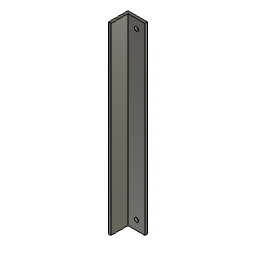
angle iron 1 inch 240 mm v12 (Autodesk Fusion 360 design; units mm, degrees)
Autodesk Fusion 360 part; units mm, degrees
sketch "Sketch1" plane through (0, 0, 0) normal (0, 0, 1) x (1, 0, 0)
  line L0 (0, 0) -> (25.4, 0)
  line L1 (0, 0) -> (0, -25.4)
  line L2 (3.175, -3.175) -> (25.4, -3.175)
  line L3 (3.175, -3.175) -> (3.175, -25.4)
  line L4 (25.4, 0) -> (25.4, -3.175)
  line L5 (0, -25.4) -> (3.175, -25.4)
  dimension "d1" = 25.4
  dimension "d2" = -3.175
  constraint coincident L0.start L1.start
  constraint horizontal L0
  constraint perpendicular L0 L1
  constraint equal L0 L1
  measures "d1" distance of L0.start L0.end
extrude "Extrude1" add sketch "Sketch1" along normal blind 240
sketch "Sketch2" plane through (0, -3.175, 0) normal (0, -1, 0) x (1, 0, 0)
  line L0 (3.175, 0) -> (25.4, 0)
  line L1 (25.4, 0) -> (25.4, 240)
  line L2 (25.4, 240) -> (3.175, 240)
  line L3 (3.175, 240) -> (3.175, 0)
  circle A0 centre (14.2875, 228) radius 2.75
  circle A1 centre (14.2875, 12) radius 2.75
  line L4 (14.2875, 240) -> (14.2875, 0) construction
  dimension "d5" = 5.5
  dimension "d6" = 12
  dimension "d7" = 12
  constraint equal A0 A1
  constraint midpoint L2 L4.start
  constraint midpoint L0 L4.end
  constraint coincident A1.centre L4
  constraint coincident A0.centre L4
  measures "d5" diameter of A0
  measures "d6" distance of L2 A0.centre
  measures "d7" distance of L0 A1.centre
hole "Hole1" at (14.2875, -3.175, 12) at (14.2875, -3.175, 228) direction (0, 1, 0) diameter 5.5 depth 7 tip angle 118
